Autodesk Fusion 360 part; units mm, degrees
(part 3 of 11)
  line L1882 (214.369, 95.2168) -> (214.369, 94.2164)
  line L1883 (214.369, 94.2164) -> (213.57, 94.2164)
  line L1884 (213.57, 94.2164) -> (213.57, 91.1172)
  line L1885 (213.57, 91.1172) -> (214.369, 91.1172)
  line L1886 (214.369, 91.1172) -> (214.369, 85.3172)
  line L1887 (214.369, 85.3172) -> (213.57, 85.3172)
  line L1888 (213.57, 85.3172) -> (213.57, 82.2166)
  line L1889 (213.57, 82.2166) -> (214.369, 82.2166)
  line L1890 (214.369, 82.2166) -> (214.369, 81.2161)
  line L1891 (214.369, 81.2161) -> (228.37, 81.2161)
  line L1892 (228.37, 81.2161) -> (228.37, 82.2166)
  line L1893 (228.37, 82.2166) -> (229.169, 82.2166)
  line L1894 (229.169, 82.2166) -> (229.169, 85.3172)
  line L1895 (229.169, 85.3172) -> (228.37, 85.3172)
  line L1896 (228.37, 85.3172) -> (228.37, 91.1172)
  line L1897 (228.37, 91.1172) -> (229.169, 91.1172)
  line L1898 (229.169, 91.1172) -> (229.169, 94.2164)
  line L1899 (229.169, 94.2164) -> (228.37, 94.2164)
  line L1900 (228.37, 94.2164) -> (228.37, 95.2168)
  line L1901 (228.37, 95.2168) -> (214.369, 95.2168)
  line L1902 (233.419, 95.2168) -> (233.419, 94.2164)
  line L1903 (233.419, 94.2164) -> (232.62, 94.2164)
  line L1904 (232.62, 94.2164) -> (232.62, 91.1172)
  line L1905 (232.62, 91.1172) -> (233.419, 91.1172)
  line L1906 (233.419, 91.1172) -> (233.419, 85.3172)
  line L1907 (233.419, 85.3172) -> (232.62, 85.3172)
  line L1908 (232.62, 85.3172) -> (232.62, 82.2166)
  line L1909 (232.62, 82.2166) -> (233.419, 82.2166)
  line L1910 (233.419, 82.2166) -> (233.419, 81.2161)
  line L1911 (233.419, 81.2161) -> (247.42, 81.2161)
  line L1912 (247.42, 81.2161) -> (247.42, 82.2166)
  line L1913 (247.42, 82.2166) -> (248.219, 82.2166)
  line L1914 (248.219, 82.2166) -> (248.219, 85.3172)
  line L1915 (248.219, 85.3172) -> (247.42, 85.3172)
  line L1916 (247.42, 85.3172) -> (247.42, 91.1172)
  line L1917 (247.42, 91.1172) -> (248.219, 91.1172)
  line L1918 (248.219, 91.1172) -> (248.219, 94.2164)
  line L1919 (248.219, 94.2164) -> (247.42, 94.2164)
  line L1920 (247.42, 94.2164) -> (247.42, 95.2168)
  line L1921 (247.42, 95.2168) -> (233.419, 95.2168)
  line L1922 (295.331, 95.2168) -> (295.331, 94.2164)
  line L1923 (295.331, 94.2164) -> (294.531, 94.2164)
  line L1924 (294.531, 94.2164) -> (294.531, 91.1172)
  line L1925 (294.531, 91.1172) -> (295.331, 91.1172)
  line L1926 (295.331, 91.1172) -> (295.331, 85.3172)
  line L1927 (295.331, 85.3172) -> (294.531, 85.3172)
  line L1928 (294.531, 85.3172) -> (294.531, 82.2166)
  line L1929 (294.531, 82.2166) -> (295.331, 82.2166)
  line L1930 (295.331, 82.2166) -> (295.331, 81.2161)
  line L1931 (295.331, 81.2161) -> (309.331, 81.2161)
  line L1932 (309.331, 81.2161) -> (309.331, 82.2166)
  line L1933 (309.331, 82.2166) -> (310.132, 82.2166)
  line L1934 (310.132, 82.2166) -> (310.132, 85.3172)
  line L1935 (310.132, 85.3172) -> (309.331, 85.3172)
  line L1936 (309.331, 85.3172) -> (309.331, 91.1172)
  line L1937 (309.331, 91.1172) -> (310.132, 91.1172)
  line L1938 (310.132, 91.1172) -> (310.132, 94.2164)
  line L1939 (310.132, 94.2164) -> (309.331, 94.2164)
  line L1940 (309.331, 94.2164) -> (309.331, 95.2168)
  line L1941 (309.331, 95.2168) -> (295.331, 95.2168)
  line L1942 (314.381, 95.2168) -> (314.381, 94.2164)
  line L1943 (314.381, 94.2164) -> (313.581, 94.2164)
  line L1944 (313.581, 94.2164) -> (313.581, 91.1172)
  line L1945 (313.581, 91.1172) -> (314.381, 91.1172)
  line L1946 (314.381, 91.1172) -> (314.381, 85.3172)
  line L1947 (314.381, 85.3172) -> (313.581, 85.3172)
  line L1948 (313.581, 85.3172) -> (313.581, 82.2166)
  line L1949 (313.581, 82.2166) -> (314.381, 82.2166)
  line L1950 (314.381, 82.2166) -> (314.381, 81.2161)
  line L1951 (314.381, 81.2161) -> (328.381, 81.2161)
  line L1952 (328.381, 81.2161) -> (328.381, 82.2166)
  line L1953 (328.381, 82.2166) -> (329.182, 82.2166)
  line L1954 (329.182, 82.2166) -> (329.182, 85.3172)
  line L1955 (329.182, 85.3172) -> (328.381, 85.3172)
  line L1956 (328.381, 85.3172) -> (328.381, 91.1172)
  line L1957 (328.381, 91.1172) -> (329.182, 91.1172)
  line L1958 (329.182, 91.1172) -> (329.182, 94.2164)
  line L1959 (329.182, 94.2164) -> (328.381, 94.2164)
  line L1960 (328.381, 94.2164) -> (328.381, 95.2168)
  line L1961 (328.381, 95.2168) -> (314.381, 95.2168)
  line L1962 (333.431, 95.2168) -> (333.431, 94.2164)
  line L1963 (333.431, 94.2164) -> (332.631, 94.2164)
  line L1964 (332.631, 94.2164) -> (332.631, 91.1172)
  line L1965 (332.631, 91.1172) -> (333.431, 91.1172)
  line L1966 (333.431, 91.1172) -> (333.431, 85.3172)
  line L1967 (333.431, 85.3172) -> (332.631, 85.3172)
  line L1968 (332.631, 85.3172) -> (332.631, 82.2166)
  line L1969 (332.631, 82.2166) -> (333.431, 82.2166)
  line L1970 (333.431, 82.2166) -> (333.431, 81.2161)
  line L1971 (333.431, 81.2161) -> (347.431, 81.2161)
  line L1972 (347.431, 81.2161) -> (347.431, 82.2166)
  line L1973 (347.431, 82.2166) -> (348.232, 82.2166)
  line L1974 (348.232, 82.2166) -> (348.232, 85.3172)
  line L1975 (348.232, 85.3172) -> (347.431, 85.3172)
  line L1976 (347.431, 85.3172) -> (347.431, 91.1172)
  line L1977 (347.431, 91.1172) -> (348.232, 91.1172)
  line L1978 (348.232, 91.1172) -> (348.232, 94.2164)
  line L1979 (348.232, 94.2164) -> (347.431, 94.2164)
  line L1980 (347.431, 94.2164) -> (347.431, 95.2168)
  line L1981 (347.431, 95.2168) -> (333.431, 95.2168)
  line L1982 (357.244, 95.2168) -> (357.244, 94.2164)
  line L1983 (357.244, 94.2164) -> (356.443, 94.2164)
  line L1984 (356.443, 94.2164) -> (356.443, 91.1172)
  line L1985 (356.443, 91.1172) -> (357.244, 91.1172)
  line L1986 (357.244, 91.1172) -> (357.244, 85.3172)
  line L1987 (357.244, 85.3172) -> (356.443, 85.3172)
  line L1988 (356.443, 85.3172) -> (356.443, 82.2166)
  line L1989 (356.443, 82.2166) -> (357.244, 82.2166)
  line L1990 (357.244, 82.2166) -> (357.244, 81.2161)
  line L1991 (357.244, 81.2161) -> (371.246, 81.2161)
  line L1992 (371.246, 81.2161) -> (371.246, 82.2166)
  line L1993 (371.246, 82.2166) -> (372.043, 82.2166)
  line L1994 (372.043, 82.2166) -> (372.043, 85.3172)
  line L1995 (372.043, 85.3172) -> (371.246, 85.3172)
  line L1996 (371.246, 85.3172) -> (371.246, 91.1172)
  line L1997 (371.246, 91.1172) -> (372.043, 91.1172)
  line L1998 (372.043, 91.1172) -> (372.043, 94.2164)
  line L1999 (372.043, 94.2164) -> (371.246, 94.2164)
  line L2000 (371.246, 94.2164) -> (371.246, 95.2168)
  line L2001 (371.246, 95.2168) -> (357.244, 95.2168)
  line L2002 (376.294, 95.2168) -> (376.294, 94.2164)
  line L2003 (376.294, 94.2164) -> (375.493, 94.2164)
  line L2004 (375.493, 94.2164) -> (375.493, 91.1172)
  line L2005 (375.493, 91.1172) -> (376.294, 91.1172)
  line L2006 (376.294, 91.1172) -> (376.294, 85.3172)
  line L2007 (376.294, 85.3172) -> (375.493, 85.3172)
  line L2008 (375.493, 85.3172) -> (375.493, 82.2166)
  line L2009 (375.493, 82.2166) -> (376.294, 82.2166)
  line L2010 (376.294, 82.2166) -> (376.294, 81.2161)
  line L2011 (376.294, 81.2161) -> (390.296, 81.2161)
  line L2012 (390.296, 81.2161) -> (390.296, 82.2166)
  line L2013 (390.296, 82.2166) -> (391.093, 82.2166)
  line L2014 (391.093, 82.2166) -> (391.093, 85.3172)
  line L2015 (391.093, 85.3172) -> (390.296, 85.3172)
  line L2016 (390.296, 85.3172) -> (390.296, 91.1172)
  line L2017 (390.296, 91.1172) -> (391.093, 91.1172)
  line L2018 (391.093, 91.1172) -> (391.093, 94.2164)
  line L2019 (391.093, 94.2164) -> (390.296, 94.2164)
  line L2020 (390.296, 94.2164) -> (390.296, 95.2168)
  line L2021 (390.296, 95.2168) -> (376.294, 95.2168)
  line L2022 (395.344, 95.2168) -> (395.344, 94.2164)
  line L2023 (395.344, 94.2164) -> (394.543, 94.2164)
  line L2024 (394.543, 94.2164) -> (394.543, 91.1172)
  line L2025 (394.543, 91.1172) -> (395.344, 91.1172)
  line L2026 (395.344, 91.1172) -> (395.344, 85.3172)
  line L2027 (395.344, 85.3172) -> (394.543, 85.3172)
  line L2028 (394.543, 85.3172) -> (394.543, 82.2166)
  line L2029 (394.543, 82.2166) -> (395.344, 82.2166)
  line L2030 (395.344, 82.2166) -> (395.344, 81.2161)
  line L2031 (395.344, 81.2161) -> (409.346, 81.2161)
  line L2032 (409.346, 81.2161) -> (409.346, 82.2166)
  line L2033 (409.346, 82.2166) -> (410.143, 82.2166)
  line L2034 (410.143, 82.2166) -> (410.143, 85.3172)
  line L2035 (410.143, 85.3172) -> (409.346, 85.3172)
  line L2036 (409.346, 85.3172) -> (409.346, 91.1172)
  line L2037 (409.346, 91.1172) -> (410.143, 91.1172)
  line L2038 (410.143, 91.1172) -> (410.143, 94.2164)
  line L2039 (410.143, 94.2164) -> (409.346, 94.2164)
  line L2040 (409.346, 94.2164) -> (409.346, 95.2168)
  line L2041 (409.346, 95.2168) -> (395.344, 95.2168)
  line L2042 (414.394, 95.2168) -> (414.394, 94.2164)
  line L2043 (414.394, 94.2164) -> (413.593, 94.2164)
  line L2044 (413.593, 94.2164) -> (413.593, 91.1172)
  line L2045 (413.593, 91.1172) -> (414.394, 91.1172)
  line L2046 (414.394, 91.1172) -> (414.394, 85.3172)
  line L2047 (414.394, 85.3172) -> (413.593, 85.3172)
  line L2048 (413.593, 85.3172) -> (413.593, 82.2166)
  line L2049 (413.593, 82.2166) -> (414.394, 82.2166)
  line L2050 (414.394, 82.2166) -> (414.394, 81.2161)
  line L2051 (414.394, 81.2161) -> (428.396, 81.2161)
  line L2052 (428.396, 81.2161) -> (428.396, 82.2166)
  line L2053 (428.396, 82.2166) -> (429.193, 82.2166)
  line L2054 (429.193, 82.2166) -> (429.193, 85.3172)
  line L2055 (429.193, 85.3172) -> (428.396, 85.3172)
  line L2056 (428.396, 85.3172) -> (428.396, 91.1172)
  line L2057 (428.396, 91.1172) -> (429.193, 91.1172)
  line L2058 (429.193, 91.1172) -> (429.193, 94.2164)
  line L2059 (429.193, 94.2164) -> (428.396, 94.2164)
  line L2060 (428.396, 94.2164) -> (428.396, 95.2168)
  line L2061 (428.396, 95.2168) -> (414.394, 95.2168)
  line L2062 (4.819, 123.793) -> (4.819, 122.793)
  line L2063 (4.819, 122.793) -> (4.0197, 122.793)
  line L2064 (4.0197, 122.793) -> (4.0197, 119.692)
  line L2065 (4.0197, 119.692) -> (4.819, 119.692)
  line L2066 (4.819, 119.692) -> (4.819, 113.892)
  line L2067 (4.819, 113.892) -> (4.0197, 113.892)
  line L2068 (4.0197, 113.892) -> (4.0197, 110.792)
  line L2069 (4.0197, 110.792) -> (4.819, 110.792)
  line L2070 (4.819, 110.792) -> (4.819, 109.791)
  line L2071 (4.819, 109.791) -> (18.8199, 109.791)
  line L2072 (18.8199, 109.791) -> (18.8199, 110.792)
  line L2073 (18.8199, 110.792) -> (19.6191, 110.792)
  line L2074 (19.6191, 110.792) -> (19.6191, 113.892)
  line L2075 (19.6191, 113.892) -> (18.8199, 113.892)
  line L2076 (18.8199, 113.892) -> (18.8199, 119.692)
  line L2077 (18.8199, 119.692) -> (19.6191, 119.692)
  line L2078 (19.6191, 119.692) -> (19.6191, 122.793)
  line L2079 (19.6191, 122.793) -> (18.8199, 122.793)
  line L2080 (18.8199, 122.793) -> (18.8199, 123.793)
  line L2081 (18.8199, 123.793) -> (4.819, 123.793)
  line L2082 (42.9189, 123.793) -> (42.9189, 122.793)
  line L2083 (42.9189, 122.793) -> (42.1199, 122.793)
  line L2084 (42.1199, 122.793) -> (42.1199, 119.692)
  line L2085 (42.1199, 119.692) -> (42.9189, 119.692)
  line L2086 (42.9189, 119.692) -> (42.9189, 113.892)
  line L2087 (42.9189, 113.892) -> (42.1199, 113.892)
  line L2088 (42.1199, 113.892) -> (42.1199, 110.792)
  line L2089 (42.1199, 110.792) -> (42.9189, 110.792)
  line L2090 (42.9189, 110.792) -> (42.9189, 109.791)
  line L2091 (42.9189, 109.791) -> (56.92, 109.791)
  line L2092 (56.92, 109.791) -> (56.92, 110.792)
  line L2093 (56.92, 110.792) -> (57.719, 110.792)
  line L2094 (57.719, 110.792) -> (57.719, 113.892)
  line L2095 (57.719, 113.892) -> (56.92, 113.892)
  line L2096 (56.92, 113.892) -> (56.92, 119.692)
  line L2097 (56.92, 119.692) -> (57.719, 119.692)
  line L2098 (57.719, 119.692) -> (57.719, 122.793)
  line L2099 (57.719, 122.793) -> (56.92, 122.793)
  line L2100 (56.92, 122.793) -> (56.92, 123.793)
  line L2101 (56.92, 123.793) -> (42.9189, 123.793)
  line L2102 (61.9689, 123.793) -> (61.9689, 122.793)
  line L2103 (61.9689, 122.793) -> (61.1699, 122.793)
  line L2104 (61.1699, 122.793) -> (61.1699, 119.692)
  line L2105 (61.1699, 119.692) -> (61.9689, 119.692)
  line L2106 (61.9689, 119.692) -> (61.9689, 113.892)
  line L2107 (61.9689, 113.892) -> (61.1699, 113.892)
  line L2108 (61.1699, 113.892) -> (61.1699, 110.792)
  line L2109 (61.1699, 110.792) -> (61.9689, 110.792)
  line L2110 (61.9689, 110.792) -> (61.9689, 109.791)
  line L2111 (61.9689, 109.791) -> (75.97, 109.791)
  line L2112 (75.97, 109.791) -> (75.97, 110.792)
  line L2113 (75.97, 110.792) -> (76.769, 110.792)
  line L2114 (76.769, 110.792) -> (76.769, 113.892)
  line L2115 (76.769, 113.892) -> (75.97, 113.892)
  line L2116 (75.97, 113.892) -> (75.97, 119.692)
  line L2117 (75.97, 119.692) -> (76.769, 119.692)
  line L2118 (76.769, 119.692) -> (76.769, 122.793)
  line L2119 (76.769, 122.793) -> (75.97, 122.793)
  line L2120 (75.97, 122.793) -> (75.97, 123.793)
  line L2121 (75.97, 123.793) -> (61.9689, 123.793)
  line L2122 (81.0189, 123.793) -> (81.0189, 122.793)
  line L2123 (81.0189, 122.793) -> (80.2199, 122.793)
  line L2124 (80.2199, 122.793) -> (80.2199, 119.692)
  line L2125 (80.2199, 119.692) -> (81.0189, 119.692)
  line L2126 (81.0189, 119.692) -> (81.0189, 113.892)
  line L2127 (81.0189, 113.892) -> (80.2199, 113.892)
  line L2128 (80.2199, 113.892) -> (80.2199, 110.792)
  line L2129 (80.2199, 110.792) -> (81.0189, 110.792)
  line L2130 (81.0189, 110.792) -> (81.0189, 109.791)
  line L2131 (81.0189, 109.791) -> (95.02, 109.791)
  line L2132 (95.02, 109.791) -> (95.02, 110.792)
  line L2133 (95.02, 110.792) -> (95.819, 110.792)
  line L2134 (95.819, 110.792) -> (95.819, 113.892)
  line L2135 (95.819, 113.892) -> (95.02, 113.892)
  line L2136 (95.02, 113.892) -> (95.02, 119.692)
  line L2137 (95.02, 119.692) -> (95.819, 119.692)
  line L2138 (95.819, 119.692) -> (95.819, 122.793)
  line L2139 (95.819, 122.793) -> (95.02, 122.793)
  line L2140 (95.02, 122.793) -> (95.02, 123.793)
  line L2141 (95.02, 123.793) -> (81.0189, 123.793)
  line L2142 (100.069, 123.793) -> (100.069, 122.793)
  line L2143 (100.069, 122.793) -> (99.2699, 122.793)
  line L2144 (99.2699, 122.793) -> (99.2699, 119.692)
  line L2145 (99.2699, 119.692) -> (100.069, 119.692)
  line L2146 (100.069, 119.692) -> (100.069, 113.892)
  line L2147 (100.069, 113.892) -> (99.2699, 113.892)
  line L2148 (99.2699, 113.892) -> (99.2699, 110.792)
  line L2149 (99.2699, 110.792) -> (100.069, 110.792)
  line L2150 (100.069, 110.792) -> (100.069, 109.791)
  line L2151 (100.069, 109.791) -> (114.07, 109.791)
  line L2152 (114.07, 109.791) -> (114.07, 110.792)
  line L2153 (114.07, 110.792) -> (114.869, 110.792)
  line L2154 (114.869, 110.792) -> (114.869, 113.892)
  line L2155 (114.869, 113.892) -> (114.07, 113.892)
  line L2156 (114.07, 113.892) -> (114.07, 119.692)
  line L2157 (114.07, 119.692) -> (114.869, 119.692)
  line L2158 (114.869, 119.692) -> (114.869, 122.793)
  line L2159 (114.869, 122.793) -> (114.07, 122.793)
  line L2160 (114.07, 122.793) -> (114.07, 123.793)
  line L2161 (114.07, 123.793) -> (100.069, 123.793)
  line L2162 (128.644, 123.793) -> (128.644, 122.793)
  line L2163 (128.644, 122.793) -> (127.845, 122.793)
  line L2164 (127.845, 122.793) -> (127.845, 119.692)
  line L2165 (127.845, 119.692) -> (128.644, 119.692)
  line L2166 (128.644, 119.692) -> (128.644, 113.892)
  line L2167 (128.644, 113.892) -> (127.845, 113.892)
  line L2168 (127.845, 113.892) -> (127.845, 110.792)
  line L2169 (127.845, 110.792) -> (128.644, 110.792)
  line L2170 (128.644, 110.792) -> (128.644, 109.791)
  line L2171 (128.644, 109.791) -> (142.645, 109.791)
  line L2172 (142.645, 109.791) -> (142.645, 110.792)
  line L2173 (142.645, 110.792) -> (143.444, 110.792)
  line L2174 (143.444, 110.792) -> (143.444, 113.892)
  line L2175 (143.444, 113.892) -> (142.645, 113.892)
  line L2176 (142.645, 113.892) -> (142.645, 119.692)
  line L2177 (142.645, 119.692) -> (143.444, 119.692)
  line L2178 (143.444, 119.692) -> (143.444, 122.793)
  line L2179 (143.444, 122.793) -> (142.645, 122.793)
  line L2180 (142.645, 122.793) -> (142.645, 123.793)
  line L2181 (142.645, 123.793) -> (128.644, 123.793)
  line L2182 (147.694, 123.793) -> (147.694, 122.793)
  line L2183 (147.694, 122.793) -> (146.895, 122.793)
  line L2184 (146.895, 122.793) -> (146.895, 119.692)
  line L2185 (146.895, 119.692) -> (147.694, 119.692)
  line L2186 (147.694, 119.692) -> (147.694, 113.892)
  line L2187 (147.694, 113.892) -> (146.895, 113.892)
  line L2188 (146.895, 113.892) -> (146.895, 110.792)
  line L2189 (146.895, 110.792) -> (147.694, 110.792)
  line L2190 (147.694, 110.792) -> (147.694, 109.791)
  line L2191 (147.694, 109.791) -> (161.695, 109.791)
  line L2192 (161.695, 109.791) -> (161.695, 110.792)
  line L2193 (161.695, 110.792) -> (162.494, 110.792)
  line L2194 (162.494, 110.792) -> (162.494, 113.892)
  line L2195 (162.494, 113.892) -> (161.695, 113.892)
  line L2196 (161.695, 113.892) -> (161.695, 119.692)
  line L2197 (161.695, 119.692) -> (162.494, 119.692)
  line L2198 (162.494, 119.692) -> (162.494, 122.793)
  line L2199 (162.494, 122.793) -> (161.695, 122.793)
  line L2200 (161.695, 122.793) -> (161.695, 123.793)
  line L2201 (161.695, 123.793) -> (147.694, 123.793)
  line L2202 (166.744, 123.793) -> (166.744, 122.793)
  line L2203 (166.744, 122.793) -> (165.945, 122.793)
  line L2204 (165.945, 122.793) -> (165.945, 119.692)
  line L2205 (165.945, 119.692) -> (166.744, 119.692)
  line L2206 (166.744, 119.692) -> (166.744, 113.892)
  line L2207 (166.744, 113.892) -> (165.945, 113.892)
  line L2208 (165.945, 113.892) -> (165.945, 110.792)
  line L2209 (165.945, 110.792) -> (166.744, 110.792)
  line L2210 (166.744, 110.792) -> (166.744, 109.791)
  line L2211 (166.744, 109.791) -> (180.745, 109.791)
  line L2212 (180.745, 109.791) -> (180.745, 110.792)
  line L2213 (180.745, 110.792) -> (181.544, 110.792)
  line L2214 (181.544, 110.792) -> (181.544, 113.892)
  line L2215 (181.544, 113.892) -> (180.745, 113.892)
  line L2216 (180.745, 113.892) -> (180.745, 119.692)
  line L2217 (180.745, 119.692) -> (181.544, 119.692)
  line L2218 (181.544, 119.692) -> (181.544, 122.793)
  line L2219 (181.544, 122.793) -> (180.745, 122.793)
  line L2220 (180.745, 122.793) -> (180.745, 123.793)
  line L2221 (180.745, 123.793) -> (166.744, 123.793)
  line L2222 (185.794, 123.793) -> (185.794, 122.793)
  line L2223 (185.794, 122.793) -> (184.995, 122.793)
  line L2224 (184.995, 122.793) -> (184.995, 119.692)
  line L2225 (184.995, 119.692) -> (185.794, 119.692)
  line L2226 (185.794, 119.692) -> (185.794, 113.892)
  line L2227 (185.794, 113.892) -> (184.995, 113.892)
  line L2228 (184.995, 113.892) -> (184.995, 110.792)
  line L2229 (184.995, 110.792) -> (185.794, 110.792)
  line L2230 (185.794, 110.792) -> (185.794, 109.791)
  line L2231 (185.794, 109.791) -> (199.795, 109.791)
  line L2232 (199.795, 109.791) -> (199.795, 110.792)
  line L2233 (199.795, 110.792) -> (200.594, 110.792)
  line L2234 (200.594, 110.792) -> (200.594, 113.892)
  line L2235 (200.594, 113.892) -> (199.795, 113.892)
  line L2236 (199.795, 113.892) -> (199.795, 119.692)
  line L2237 (199.795, 119.692) -> (200.594, 119.692)
  line L2238 (200.594, 119.692) -> (200.594, 122.793)
  line L2239 (200.594, 122.793) -> (199.795, 122.793)
  line L2240 (199.795, 122.793) -> (199.795, 123.793)
  line L2241 (199.795, 123.793) -> (185.794, 123.793)
  line L2242 (214.369, 123.793) -> (214.369, 122.793)
  line L2243 (214.369, 122.793) -> (213.57, 122.793)
  line L2244 (213.57, 122.793) -> (213.57, 119.692)
  line L2245 (213.57, 119.692) -> (214.369, 119.692)
  line L2246 (214.369, 119.692) -> (214.369, 113.892)
  line L2247 (214.369, 113.892) -> (213.57, 113.892)
  line L2248 (213.57, 113.892) -> (213.57, 110.792)
  line L2249 (213.57, 110.792) -> (214.369, 110.792)
  line L2250 (214.369, 110.792) -> (214.369, 109.791)
  line L2251 (214.369, 109.791) -> (228.37, 109.791)
  line L2252 (228.37, 109.791) -> (228.37, 110.792)
  line L2253 (228.37, 110.792) -> (229.169, 110.792)
  line L2254 (229.169, 110.792) -> (229.169, 113.892)
  line L2255 (229.169, 113.892) -> (228.37, 113.892)
  line L2256 (228.37, 113.892) -> (228.37, 119.692)
  line L2257 (228.37, 119.692) -> (229.169, 119.692)
  line L2258 (229.169, 119.692) -> (229.169, 122.793)
  line L2259 (229.169, 122.793) -> (228.37, 122.793)
  line L2260 (228.37, 122.793) -> (228.37, 123.793)
  line L2261 (228.37, 123.793) -> (214.369, 123.793)
  line L2262 (233.419, 123.793) -> (233.419, 122.793)
  line L2263 (233.419, 122.793) -> (232.62, 122.793)
  line L2264 (232.62, 122.793) -> (232.62, 119.692)
  line L2265 (232.62, 119.692) -> (233.419, 119.692)
  line L2266 (233.419, 119.692) -> (233.419, 113.892)
  line L2267 (233.419, 113.892) -> (232.62, 113.892)
  line L2268 (232.62, 113.892) -> (232.62, 110.792)
  line L2269 (232.62, 110.792) -> (233.419, 110.792)
  line L2270 (233.419, 110.792) -> (233.419, 109.791)
  line L2271 (233.419, 109.791) -> (247.42, 109.791)
  line L2272 (247.42, 109.791) -> (247.42, 110.792)
  line L2273 (247.42, 110.792) -> (248.219, 110.792)
  line L2274 (248.219, 110.792) -> (248.219, 113.892)
  line L2275 (248.219, 113.892) -> (247.42, 113.892)
  line L2276 (247.42, 113.892) -> (247.42, 119.692)
  line L2277 (247.42, 119.692) -> (248.219, 119.692)
  line L2278 (248.219, 119.692) -> (248.219, 122.793)
  line L2279 (248.219, 122.793) -> (247.42, 122.793)
  line L2280 (247.42, 122.793) -> (247.42, 123.793)
  line L2281 (247.42, 123.793) -> (233.419, 123.793)
  line L2282 (252.469, 123.793) -> (252.469, 122.793)
  line L2283 (252.469, 122.793) -> (251.67, 122.793)
  line L2284 (251.67, 122.793) -> (251.67, 119.692)
  line L2285 (251.67, 119.692) -> (252.469, 119.692)
  line L2286 (252.469, 119.692) -> (252.469, 113.892)
  line L2287 (252.469, 113.892) -> (251.67, 113.892)
  line L2288 (251.67, 113.892) -> (251.67, 110.792)
  line L2289 (251.67, 110.792) -> (252.469, 110.792)
  line L2290 (252.469, 110.792) -> (252.469, 109.791)
  line L2291 (252.469, 109.791) -> (266.47, 109.791)
  line L2292 (266.47, 109.791) -> (266.47, 110.792)
  line L2293 (266.47, 110.792) -> (267.269, 110.792)
  line L2294 (267.269, 110.792) -> (267.269, 113.892)
  line L2295 (267.269, 113.892) -> (266.47, 113.892)
  line L2296 (266.47, 113.892) -> (266.47, 119.692)
  line L2297 (266.47, 119.692) -> (267.269, 119.692)
  line L2298 (267.269, 119.692) -> (267.269, 122.793)
  line L2299 (267.269, 122.793) -> (266.47, 122.793)
  line L2300 (266.47, 122.793) -> (266.47, 123.793)
  line L2301 (266.47, 123.793) -> (252.469, 123.793)
  line L2302 (271.519, 123.793) -> (271.519, 122.793)
  line L2303 (271.519, 122.793) -> (270.72, 122.793)
  line L2304 (270.72, 122.793) -> (270.72, 119.692)
  line L2305 (270.72, 119.692) -> (271.519, 119.692)
  line L2306 (271.519, 119.692) -> (271.519, 113.892)
  line L2307 (271.519, 113.892) -> (270.72, 113.892)
  line L2308 (270.72, 113.892) -> (270.72, 110.792)
  line L2309 (270.72, 110.792) -> (271.519, 110.792)
  line L2310 (271.519, 110.792) -> (271.519, 109.791)
  line L2311 (271.519, 109.791) -> (285.52, 109.791)
  line L2312 (285.52, 109.791) -> (285.52, 110.792)
  line L2313 (285.52, 110.792) -> (286.319, 110.792)
  line L2314 (286.319, 110.792) -> (286.319, 113.892)
  line L2315 (286.319, 113.892) -> (285.52, 113.892)
  line L2316 (285.52, 113.892) -> (285.52, 119.692)
  line L2317 (285.52, 119.692) -> (286.319, 119.692)
  line L2318 (286.319, 119.692) -> (286.319, 122.793)
  line L2319 (286.319, 122.793) -> (285.52, 122.793)
  line L2320 (285.52, 122.793) -> (285.52, 123.793)
  line L2321 (285.52, 123.793) -> (271.519, 123.793)
  line L2322 (295.331, 123.793) -> (295.331, 122.793)
  line L2323 (295.331, 122.793) -> (294.531, 122.793)
  line L2324 (294.531, 122.793) -> (294.531, 119.692)
  line L2325 (294.531, 119.692) -> (295.331, 119.692)
  line L2326 (295.331, 119.692) -> (295.331, 113.892)
  line L2327 (295.331, 113.892) -> (294.531, 113.892)
  line L2328 (294.531, 113.892) -> (294.531, 110.792)
  line L2329 (294.531, 110.792) -> (295.331, 110.792)
  line L2330 (295.331, 110.792) -> (295.331, 109.791)
  line L2331 (295.331, 109.791) -> (309.331, 109.791)
  line L2332 (309.331, 109.791) -> (309.331, 110.792)
  line L2333 (309.331, 110.792) -> (310.132, 110.792)
  line L2334 (310.132, 110.792) -> (310.132, 113.892)
  line L2335 (310.132, 113.892) -> (309.331, 113.892)
  line L2336 (309.331, 113.892) -> (309.331, 119.692)
  line L2337 (309.331, 119.692) -> (310.132, 119.692)
  line L2338 (310.132, 119.692) -> (310.132, 122.793)
  line L2339 (310.132, 122.793) -> (309.331, 122.793)
  line L2340 (309.331, 122.793) -> (309.331, 123.793)
  line L2341 (309.331, 123.793) -> (295.331, 123.793)
  line L2342 (314.381, 123.793) -> (314.381, 122.793)
  line L2343 (314.381, 122.793) -> (313.581, 122.793)
  line L2344 (313.581, 122.793) -> (313.581, 119.692)
  line L2345 (313.581, 119.692) -> (314.381, 119.692)
  line L2346 (314.381, 119.692) -> (314.381, 113.892)
  line L2347 (314.381, 113.892) -> (313.581, 113.892)
  line L2348 (313.581, 113.892) -> (313.581, 110.792)
  line L2349 (313.581, 110.792) -> (314.381, 110.792)
  line L2350 (314.381, 110.792) -> (314.381, 109.791)
  line L2351 (314.381, 109.791) -> (328.381, 109.791)
  line L2352 (328.381, 109.791) -> (328.381, 110.792)
  line L2353 (328.381, 110.792) -> (329.182, 110.792)
  line L2354 (329.182, 110.792) -> (329.182, 113.892)
  line L2355 (329.182, 113.892) -> (328.381, 113.892)
  line L2356 (328.381, 113.892) -> (328.381, 119.692)
  line L2357 (328.381, 119.692) -> (329.182, 119.692)
  line L2358 (329.182, 119.692) -> (329.182, 122.793)
  line L2359 (329.182, 122.793) -> (328.381, 122.793)
  line L2360 (328.381, 122.793) -> (328.381, 123.793)
  line L2361 (328.381, 123.793) -> (314.381, 123.793)
  line L2362 (333.431, 123.793) -> (333.431, 122.793)
  line L2363 (333.431, 122.793) -> (332.631, 122.793)
  line L2364 (332.631, 122.793) -> (332.631, 119.692)
  line L2365 (332.631, 119.692) -> (333.431, 119.692)
  line L2366 (333.431, 119.692) -> (333.431, 113.892)
  line L2367 (333.431, 113.892) -> (332.631, 113.892)
  line L2368 (332.631, 113.892) -> (332.631, 110.792)
  line L2369 (332.631, 110.792) -> (333.431, 110.792)
  line L2370 (333.431, 110.792) -> (333.431, 109.791)
  line L2371 (333.431, 109.791) -> (347.431, 109.791)
  line L2372 (347.431, 109.791) -> (347.431, 110.792)
  line L2373 (347.431, 110.792) -> (348.232, 110.792)
  line L2374 (348.232, 110.792) -> (348.232, 113.892)
  line L2375 (348.232, 113.892) -> (347.431, 113.892)
  line L2376 (347.431, 113.892) -> (347.431, 119.692)
  line L2377 (347.431, 119.692) -> (348.232, 119.692)
  line L2378 (348.232, 119.692) -> (348.232, 122.793)
  line L2379 (348.232, 122.793) -> (347.431, 122.793)
  line L2380 (347.431, 122.793) -> (347.431, 123.793)
  line L2381 (347.431, 123.793) -> (333.431, 123.793)
  circle A0 centre (76.263, -3.2098) radius 1.7
  circle A1 centre (190.262, -3.2098) radius 1.7
  circle A2 centre (19.2003, -3.2098) radius 1.7
  circle A3 centre (271.138, -3.2098) radius 1.7
  circle A4 centre (343.137, -3.2098) radius 1.7
  circle A5 centre (407.431, -3.2098) radius 1.7
  circle A6 centre (19.2005, 131.716) radius 1.7
  circle A7 centre (76.263, 131.716) radius 1.7
  circle A8 centre (190.262, 131.716) radius 1.7
  circle A9 centre (271.138, 131.716) radius 1.7
  circle A10 centre (343.137, 131.716) radius 1.7
  circle A11 centre (407.431, 131.716) radius 1.7
  line L2382 (7.5005, 133.116) -> (7.5005, 130.316)
  line L2383 (25.9005, 133.116) -> (25.9005, 130.316)
  line L2384 (87.963, 133.116) -> (87.963, 130.316)
  line L2385 (64.563, 133.116) -> (64.563, 130.316)
  line L2386 (201.962, 133.116) -> (201.962, 130.316)
  line L2387 (178.562, 133.116) -> (178.562, 130.316)
  line L2388 (282.838, 133.116) -> (282.838, 130.316)
  line L2389 (259.438, 133.116) -> (259.438, 130.316)
  line L2390 (354.837, 133.116) -> (354.837, 130.316)
  line L2391 (331.437, 133.116) -> (331.437, 130.316)
  line L2392 (419.131, 133.116) -> (419.131, 130.316)
  line L2393 (395.731, 133.116) -> (395.731, 130.316)
  line L2394 (25.9003, -4.6098) -> (25.9003, -1.8098)
  line L2395 (7.5003, -4.6098) -> (7.5003, -1.8098)
  line L2396 (64.563, -4.6098) -> (64.563, -1.8098)
  line L2397 (87.963, -4.6098) -> (87.963, -1.8098)
  line L2398 (201.962, -4.6098) -> (201.962, -1.8098)
  line L2399 (178.562, -4.6098) -> (178.562, -1.8098)
  line L2400 (282.838, -4.6098) -> (282.838, -1.8098)
  line L2401 (259.438, -4.6098) -> (259.438, -1.8098)
  line L2402 (354.837, -4.6098) -> (354.837, -1.8098)
  line L2403 (331.437, -4.6098) -> (331.437, -1.8098)
  line L2404 (419.131, -4.6098) -> (419.131, -1.8098)
  line L2405 (395.731, -4.6098) -> (395.731, -1.8098)
  line L2406 (23.9005, 135.116) -> (9.5005, 135.116)
  line L2407 (85.963, 135.116) -> (66.563, 135.116)
  line L2408 (199.962, 135.116) -> (180.562, 135.116)
  line L2409 (280.838, 135.116) -> (261.438, 135.116)
  line L2410 (417.131, 135.116) -> (397.731, 135.116)
  line L2411 (352.837, 135.116) -> (333.437, 135.116)
  line L2412 (397.731, -6.6098) -> (417.131, -6.6098)
  line L2413 (333.437, -6.6098) -> (352.837, -6.6098)
  line L2414 (261.438, -6.6098) -> (280.838, -6.6098)
  line L2415 (180.562, -6.6098) -> (199.962, -6.6098)
  line L2416 (9.5003, -6.6098) -> (23.9003, -6.6098)
  line L2417 (66.563, -6.6098) -> (85.963, -6.6098)
  line L2418 (5.5003, 0.1902) -> (0.0951, 0.1902)
  line L2419 (62.563, 0.1902) -> (27.9003, 0.1902)
  line L2420 (176.562, 0.1902) -> (89.963, 0.1902)
  line L2421 (257.438, 0.1902) -> (203.962, 0.1902)
  line L2422 (329.437, 0.1902) -> (284.838, 0.1902)
  line L2423 (432.82, 0.1902) -> (421.131, 0.1902)
  line L2424 (393.731, 0.1902) -> (356.837, 0.1902)
  line L2425 (421.131, 128.316) -> (432.82, 128.316)
  line L2426 (356.837, 128.316) -> (393.731, 128.316)
  line L2427 (284.838, 128.316) -> (329.437, 128.316)
  line L2428 (203.962, 128.316) -> (257.438, 128.316)
  line L2429 (89.963, 128.316) -> (176.562, 128.316)
  line L2430 (0.0951, 128.316) -> (5.5005, 128.316)
  line L2431 (27.9005, 128.316) -> (62.563, 128.316)
  arc A12 (7.5003, -1.8098) -> (5.5003, 0.1902) centre (5.5003, -1.8098) ccw
  arc A13 (7.5003, -4.6098) -> (9.5003, -6.6098) centre (9.5003, -4.6098) ccw
  arc A14 (23.9003, -6.6098) -> (25.9003, -4.6098) centre (23.9003, -4.6098) ccw
  arc A15 (27.9003, 0.1902) -> (25.9003, -1.8098) centre (27.9003, -1.8098) ccw
  arc A16 (64.563, -1.8098) -> (62.563, 0.1902) centre (62.563, -1.8098) ccw
  arc A17 (64.563, -4.6098) -> (66.563, -6.6098) centre (66.563, -4.6098) ccw
  arc A18 (85.963, -6.6098) -> (87.963, -4.6098) centre (85.963, -4.6098) ccw
  arc A19 (89.963, 0.1902) -> (87.963, -1.8098) centre (89.963, -1.8098) ccw
  arc A20 (178.562, -1.8098) -> (176.562, 0.1902) centre (176.562, -1.8098) ccw
  arc A21 (178.562, -4.6098) -> (180.562, -6.6098) centre (180.562, -4.6098) ccw
  arc A22 (199.962, -6.6098) -> (201.962, -4.6098) centre (199.962, -4.6098) ccw
  arc A23 (203.962, 0.1902) -> (201.962, -1.8098) centre (203.962, -1.8098) ccw
  arc A24 (259.438, -1.8098) -> (257.438, 0.1902) centre (257.438, -1.8098) ccw
  arc A25 (259.438, -4.6098) -> (261.438, -6.6098) centre (261.438, -4.6098) ccw
  arc A26 (280.838, -6.6098) -> (282.838, -4.6098) centre (280.838, -4.6098) ccw
  arc A27 (284.838, 0.1902) -> (282.838, -1.8098) centre (284.838, -1.8098) ccw
  arc A28 (331.437, -1.8098) -> (329.437, 0.1902) centre (329.437, -1.8098) ccw
  arc A29 (331.437, -4.6098) -> (333.437, -6.6098) centre (333.437, -4.6098) ccw
  arc A30 (352.837, -6.6098) -> (354.837, -4.6098) centre (352.837, -4.6098) ccw
  arc A31 (356.837, 0.1902) -> (354.837, -1.8098) centre (356.837, -1.8098) ccw
  arc A32 (395.731, -1.8098) -> (393.731, 0.1902) centre (393.731, -1.8098) ccw
  arc A33 (395.731, -4.6098) -> (397.731, -6.6098) centre (397.731, -4.6098) ccw
  arc A34 (417.131, -6.6098) -> (419.131, -4.6098) centre (417.131, -4.6098) ccw
  arc A35 (421.131, 0.1902) -> (419.131, -1.8098) centre (421.131, -1.8098) ccw
  arc A36 (419.131, 130.316) -> (421.131, 128.316) centre (421.131, 130.316) ccw
  arc A37 (419.131, 133.116) -> (417.131, 135.116) centre (417.131, 133.116) ccw
  arc A38 (397.731, 135.116) -> (395.731, 133.116) centre (397.731, 133.116) ccw
  arc A39 (393.731, 128.316) -> (395.731, 130.316) centre (393.731, 130.316) ccw
  arc A40 (354.837, 130.316) -> (356.837, 128.316) centre (356.837, 130.316) ccw
  arc A41 (354.837, 133.116) -> (352.837, 135.116) centre (352.837, 133.116) ccw
  arc A42 (333.437, 135.116) -> (331.437, 133.116) centre (333.437, 133.116) ccw
  arc A43 (329.437, 128.316) -> (331.437, 130.316) centre (329.437, 130.316) ccw
  arc A44 (282.838, 130.316) -> (284.838, 128.316) centre (284.838, 130.316) ccw
  arc A45 (282.838, 133.116) -> (280.838, 135.116) centre (280.838, 133.116) ccw
  arc A46 (261.438, 135.116) -> (259.438, 133.116) centre (261.438, 133.116) ccw
  arc A47 (257.438, 128.316) -> (259.438, 130.316) centre (257.438, 130.316) ccw
  arc A48 (201.962, 130.316) -> (203.962, 128.316) centre (203.962, 130.316) ccw
  arc A49 (201.962, 133.116) -> (199.962, 135.116) centre (199.962, 133.116) ccw
  arc A50 (180.562, 135.116) -> (178.562, 133.116) centre (180.562, 133.116) ccw
  arc A51 (176.562, 128.316) -> (178.562, 130.316) centre (176.562, 130.316) ccw
  arc A52 (87.963, 130.316) -> (89.963, 128.316) centre (89.963, 130.316) ccw
  arc A53 (87.963, 133.116) -> (85.963, 135.116) centre (85.963, 133.116) ccw
  arc A54 (66.563, 135.116) -> (64.563, 133.116) centre (66.563, 133.116) ccw
  arc A55 (62.563, 128.316) -> (64.563, 130.316) centre (62.563, 130.316) ccw
  arc A56 (25.9005, 130.316) -> (27.9005, 128.316) centre (27.9005, 130.316) ccw
  arc A57 (25.9005, 133.116) -> (23.9005, 135.116) centre (23.9005, 133.116) ccw
  arc A58 (9.5005, 135.116) -> (7.5005, 133.116) centre (9.5005, 133.116) ccw
  arc A59 (5.5005, 128.316) -> (7.5005, 130.316) centre (5.5005, 130.316) ccw
  line L2432 (-369.672, -123.515) -> (-369.672, -110.515)
  line L2433 (-369.172, -111.015) -> (-369.172, -123.015)
  line L2434 (-369.672, -110.515) -> (-356.972, -110.515)
  line L2435 (-356.972, -110.515) -> (-356.972, -123.515)
  line L2436 (-357.472, -111.015) -> (-369.172, -111.015)
  line L2437 (-357.472, -123.015) -> (-357.472, -111.015)
  line L2438 (-369.172, -123.015) -> (-357.472, -123.015)
  line L2439 (-356.972, -123.515) -> (-369.672, -123.515)
  line L2440 (357.472, 123.015) -> (369.172, 123.015)
  line L2441 (369.172, 123.015) -> (369.172, 111.015)
  line L2442 (369.172, 111.015) -> (357.472, 111.015)
  line L2443 (357.472, 111.015) -> (357.472, 123.015)
  line L2444 (356.972, 123.515) -> (369.672, 123.515)
  line L2445 (369.672, 123.515) -> (369.672, 110.515)
  line L2446 (369.672, 110.515) -> (356.972, 110.515)
  line L2447 (356.972, 110.515) -> (356.972, 123.515)
  dimension "d2" = 3.4
  dimension "d3" = 3.4
  dimension "d4" = 50
  dimension "d5" = 3.4
  dimension "d6" = 50
  dimension "d7" = 3.4
  dimension "d8" = 3.4
  dimension "d11" = 3.4
  dimension "d12" = 3.4
  dimension "d13" = 2
  dimension "d14" = 3.4
  dimension "d15" = 3.4
  dimension "d16" = 60
  dimension "d17" = 3.4
  dimension "d18" = 3.4
  dimension "d19" = 60
  dimension "d20" = 3.4
  dimension "d21" = 3.4
  dimension "d22" = 3.4
  dimension "d23" = 3.4
  dimension "d24" = 3.4
  dimension "d25" = 3.4
  dimension "d26" = 3.4
  dimension "d27" = 3.4
  dimension "d28" = 3.4
  dimension "d29" = 3.4
  dimension "d30" = 3.4
  dimension "d32" = 3.4
  dimension "d37" = 3.4
  dimension "d38" = 3.4
  dimension "d106" = 11.7
  dimension "d107" = 11.7
  dimension "d108" = 11.7
  dimension "d109" = 11.7
  dimension "d110" = 11.7
  dimension "d111" = 11.7
  dimension "d112" = 11.7
  dimension "d113" = 11.7
  dimension "d114" = 11.7
  dimension "d115" = 11.7
  dimension "d116" = 11.7
  dimension "d117" = 11.7
  dimension "d118" = 11.7
  dimension "d119" = 11.7
  dimension "d120" = 11.7
  dimension "d121" = 11.7
  dimension "d122" = 11.7
  dimension "d123" = 11.7
  dimension "d124" = 11.7
  dimension "d125" = 11.7
  dimension "d128" = 2
  dimension "d132" = 12
  dimension "d133" = 11.7
  dimension "d134" = 0.5
  dimension "d135" = 0.5
  dimension "d136" = 0.5
  dimension "d137" = 0.5
  dimension "d147" = 12
  dimension "d148" = 11.7
  dimension "d149" = 0.5
  dimension "d150" = 0.5
  dimension "d151" = 0.5
  dimension "d152" = 0.5
  dimension "d153" = 9.541
  dimension "d154" = 4.801
  dimension "d157" = 11.7
  dimension "d159" = 11.7
  constraint horizontal L2416
  constraint horizontal L2410
  constraint perpendicular L2382 L2430
  constraint perpendicular L2383 L2431
  constraint perpendicular L2394 L2419
  constraint perpendicular L2395 L2418
  constraint collinear L2406 L2407
  constraint collinear L2407 L2408
  constraint collinear L2408 L2409
  constraint collinear L2409 L2411
  constraint collinear L2410 L2411
  constraint collinear L2412 L2413
  constraint collinear L2413 L2414
  constraint collinear L2414 L2415
  constraint collinear L2415 L2417
  constraint collinear L2416 L2417
  constraint collinear L2418 L2419
  constraint collinear L2419 L2420
  constraint collinear L2420 L2421
  constraint collinear L2421 L2422
  constraint collinear L2422 L2424
  constraint collinear L2423 L2424
  constraint collinear L2425 L2426
  constraint collinear L2426 L2427
  constraint collinear L2427 L2429
  constraint perpendicular L2389 L2428
  constraint collinear L2429 L2431
  constraint collinear L2430 L2431
  constraint tangent L2395 A12
  constraint tangent L2418 A12
  constraint tangent L2395 A13
  constraint tangent L2416 A13
  constraint equal A12 A13
  constraint tangent L2416 A14
  constraint tangent L2394 A14
  constraint equal A12 A14
  constraint tangent L2394 A15
  constraint tangent L2419 A15
  constraint equal A12 A15
  constraint tangent L2419 A16
  constraint tangent L2396 A16
  constraint equal A12 A16
  constraint tangent L2396 A17
  constraint tangent L2417 A17
  constraint equal A12 A17
  constraint tangent L2417 A18
  constraint tangent L2397 A18
  constraint equal A12 A18
  constraint tangent L2397 A19
  constraint tangent L2420 A19
  constraint equal A12 A19
  constraint tangent L2420 A20
  constraint tangent L2399 A20
  constraint equal A12 A20
  constraint tangent L2399 A21
  constraint tangent L2415 A21
  constraint equal A12 A21
  constraint tangent L2415 A22
  constraint tangent L2398 A22
  constraint equal A12 A22
  constraint tangent L2398 A23
  constraint tangent L2421 A23
  constraint equal A12 A23
  constraint tangent L2421 A24
  constraint tangent L2401 A24
  constraint equal A12 A24
  constraint tangent L2401 A25
  constraint tangent L2414 A25
  constraint equal A12 A25
  constraint tangent L2414 A26
  constraint tangent L2400 A26
  constraint equal A12 A26
  constraint tangent L2400 A27
  constraint tangent L2422 A27
  constraint equal A12 A27
  constraint tangent L2422 A28
  constraint tangent L2403 A28
  constraint equal A12 A28
  constraint tangent L2403 A29
  constraint tangent L2413 A29
  constraint equal A12 A29
  constraint tangent L2413 A30
  constraint tangent L2402 A30
  constraint equal A12 A30
  constraint tangent L2402 A31
  constraint tangent L2424 A31
  constraint equal A12 A31
  constraint tangent L2424 A32
  constraint tangent L2405 A32
  constraint equal A12 A32
  constraint tangent L2405 A33
  constraint tangent L2412 A33
  constraint equal A12 A33
  constraint tangent L2404 A34
  constraint tangent L2412 A34
  constraint equal A12 A34
  constraint tangent L2404 A35
  constraint tangent L2423 A35
  constraint equal A12 A35
  constraint tangent L2392 A36
  constraint tangent L2425 A36
  constraint equal A12 A36
  constraint tangent L2392 A37
  constraint tangent L2410 A37
  constraint equal A12 A37
  constraint tangent L2393 A38
  constraint tangent L2410 A38
  constraint equal A12 A38
  constraint tangent L2393 A39
  constraint tangent L2426 A39
  constraint equal A12 A39
  constraint tangent L2390 A40
  constraint tangent L2426 A40
  constraint equal A12 A40
  constraint tangent L2390 A41
  constraint tangent L2411 A41
  constraint equal A12 A41
  constraint tangent L2391 A42
  constraint tangent L2411 A42
  constraint equal A12 A42
  constraint tangent L2391 A43
  constraint tangent L2427 A43
  constraint equal A12 A43
  constraint tangent L2388 A44
  constraint tangent L2427 A44
  constraint equal A12 A44
  constraint tangent L2388 A45
  constraint tangent L2409 A45
  constraint equal A12 A45
  constraint tangent L2389 A46
  constraint tangent L2409 A46
  constraint equal A12 A46
  constraint tangent L2389 A47
  constraint tangent L2428 A47
  constraint equal A12 A47
  constraint tangent L2386 A48
  constraint tangent L2428 A48
  constraint equal A12 A48
  constraint tangent L2386 A49
  constraint tangent L2408 A49
  constraint equal A12 A49
  constraint tangent L2387 A50
  constraint tangent L2408 A50
  constraint equal A12 A50
  constraint tangent L2387 A51
  constraint tangent L2429 A51
  constraint equal A12 A51
  constraint tangent L2384 A52
  constraint tangent L2429 A52
  constraint equal A12 A52
  constraint tangent L2384 A53
  constraint tangent L2407 A53
  constraint equal A12 A53
  constraint tangent L2385 A54
  constraint tangent L2407 A54
  constraint equal A12 A54
  constraint tangent L2385 A55
  constraint tangent L2431 A55
  constraint equal A12 A55
  constraint tangent L2383 A56
  constraint tangent L2431 A56
  constraint equal A12 A56
  constraint tangent L2383 A57
  constraint tangent L2406 A57
  constraint equal A12 A57
  constraint tangent L2382 A58
  constraint tangent L2406 A58
  constraint equal A12 A58
  constraint tangent L2382 A59
  constraint tangent L2430 A59
  constraint equal A12 A59
  constraint horizontal L2436
  constraint vertical L2433
  constraint horizontal L2438
  constraint vertical L2437
  constraint horizontal L2439
  constraint vertical L2432
  constraint horizontal L2434
  constraint vertical L2435
  constraint horizontal L2440
  constraint vertical L2441
  constraint horizontal L2442
  constraint vertical L2443
  constraint horizontal L2444
  constraint vertical L2445
  constraint horizontal L2446
  constraint vertical L2447
  measures "d2" diameter of A0
  measures "d3" diameter of A1
  measures "d4" distance of L32 A1.centre
  measures "d5" distance of A1.centre L2421
  measures "d6" distance of L30 A0.centre
  measures "d7" distance of A0.centre L2419
  measures "d8" diameter of A2
  measures "d11" distance of A2.centre L2419
  measures "d12" diameter of A3
  measures "d13" distance of L246 A3.centre
  measures "d14" distance of A3.centre L2422
  measures "d15" diameter of A4
  measures "d16" distance of L256 A4.centre
  measures "d17" distance of A4.centre L2424
  measures "d18" diameter of A5
  measures "d19" distance of L316 A5.centre
  measures "d20" distance of A5.centre L2423
  measures "d21" diameter of A6
  measures "d22" diameter of A7
  measures "d23" diameter of A8
  measures "d24" diameter of A9
  measures "d25" diameter of A10
  measures "d26" diameter of A11
  measures "d27" distance of A11.centre L2426
  measures "d28" distance of A10.centre L2427
  measures "d29" distance of A9.centre L2427
  measures "d30" distance of A8.centre L2429
  measures "d32" distance of A6.centre L2430
  measures "d37" distance of A5.centre L2412
  measures "d38" distance of A6.centre L2406
  measures "d106" distance of A7.centre L2385
  measures "d107" distance of A7.centre L2384
  measures "d108" distance of A8.centre L2387
  measures "d109" distance of A8.centre L2386
  measures "d110" distance of A9.centre L2389
  measures "d111" distance of A9.centre L2388
  measures "d112" distance of A10.centre L2391
  measures "d113" distance of A10.centre L2390
  measures "d114" distance of A11.centre L2393
  measures "d115" distance of A11.centre L2392
  measures "d116" distance of A5.centre L2404
  measures "d117" distance of A5.centre L2405
  measures "d118" distance of A4.centre L2402
  measures "d119" distance of A4.centre L2403
  measures "d120" distance of A3.centre L2400
  measures "d121" distance of A3.centre L2401
  measures "d122" distance of A1.centre L2398
  measures "d123" distance of A1.centre L2399
  measures "d124" distance of A0.centre L2397
  measures "d125" distance of A0.centre L2396
  measures "d128" radius of A12
  measures "d132" distance of L2436 L2438
  measures "d133" distance of L2433 L2437
  measures "d134" distance of L2435 L2437
  measures "d135" distance of L2438 L2439
  measures "d136" distance of L2432 L2433
  measures "d137" distance of L2434 L2436
  measures "d147" distance of L2440 L2442
  measures "d148" distance of L2441 L2443
  measures "d149" distance of L2440 L2444
  measures "d150" distance of L2443 L2447
  measures "d151" distance of L2442 L2446
  measures "d152" distance of L2441 L2445
  measures "d153" distance of L2376 L2447
  measures "d154" distance of L2426 L2444
  measures "d157" distance of A6.centre L2382
  measures "d159" distance of A2.centre L2395
extrude "Extrude9" add sketch "Sketch2" along normal blind 1.5 contours L0 L1 L2382 L2383 L2384 L2385 L2386 L2387 L2388 L2389 L2390 L2391 L2392 L2393 L2394 L2395 L2396 L2397 L2398 L2399 L2400 L2401 L2402 L2403 L2404 L2405 L2406 L2407 L2408 L2409 L2410 L2411 L2412 L2413 L2414 L2415 L2416 L2417 L2418 L2419 L2420 L2421 L2422 L2423 L2424 L2425 L2426 L2427 L2428 L2429 L2430 L2431 A12 A13 A14 A15 A16 A17 A18 A19 A20 A21 A22 A23 A24 A25 A26 A27 A28 A29 A30 A31 A32 A33 A34 A35 A36 A37 A38 A39 A40 A41 A42 A43 A44 A45 A46 A47 A48 A49 A50 A51 A52 A53 A54 A55 A56 A57 A58 A59

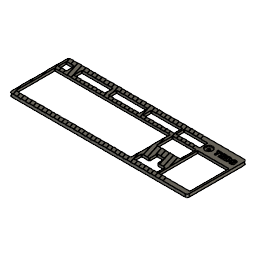
design "Top"
part number: 2026-01-27-17-33-11-118
Autodesk Fusion 360 part; units mm, degrees